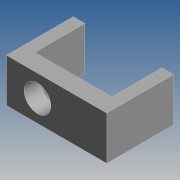
# Autodesk Inventor part: support_Servo
Saved by Autodesk Inventor 2017 (Build 210142000, 142)
## iProperties
Created: 2018-10-05
Part Number: support_Servo
Material: Générique
Document SubType Name: Modeling
Designer: Gilles Mottiez
Density: 1 g/cm^3
Appearance: Par défaut
Author: Gilles Mottiez
Autodesk Inventor part; units mm, degrees
ref_plane "YZ Plane" through (0, 0, 0) normal (1, 0, 0) x (0, 1, 0)
ref_plane "XZ Plane" through (0, 0, 0) normal (0, 1, 0) x (-1, 0, 0)
ref_plane "XY Plane" through (0, 0, 0) normal (0, 0, 1) x (1, 0, 0)
sketch "Sketch1" plane through (0, 0, 0) normal (0, 0, 1) x (1, 0, 0)
  line L0 (0, 0) -> (30, 0) construction
  line L1 (30, 0) -> (30, -20) construction
  line L2 (30, -20) -> (0, -20) construction
  line L3 (0, -20) -> (0, 0) construction
  line L4 (3.5, 0) -> (26.5, 0) construction
  line L5 (26.5, 0) -> (26.5, -15) construction
  line L6 (26.5, -15) -> (3.5, -15) construction
  line L7 (3.5, -15) -> (3.5, 0) construction
  line L8 (3.5, 0) -> (0, 0)
  line L9 (0, 0) -> (0, -20)
  line L10 (0, -20) -> (30, -20)
  line L11 (30, -20) -> (30, 0)
  line L12 (30, 0) -> (26.5, 0)
  line L13 (26.5, 0) -> (26.5, -15)
  line L14 (26.5, -15) -> (3.5, -15)
  line L15 (3.5, -15) -> (3.5, 0)
  point P0 (15, -15)
  point P1 (15, 0)
  dimension "d0" = 30
  dimension "d1" = 20
  dimension "d2" = 23
  dimension "d3" = 15
  constraints: 32 end point, 6 collinear, 4 parallel, 4 perpendicular, 2 horizontal, 2 midpoint, 1 point on line, 1 vertical alignment
  measures "d0" distance of L0.start L0.end
  measures "d1" distance of L2.end L0.start
  measures "d2" distance of L5.end L6.end
  measures "d3" distance of L4.end L5.end
extrude "Extrusion1" add sketch "Sketch1" along normal blind 13
sketch "Esquisse2" plane through (3.5, -15, 0) normal (0, 1, 0) x (1, 0, 0)
  line L0 (0, 0) -> (23, 0) construction
  line L1 (0, 0) -> (0, -13) construction
  line L2 (23, -13) -> (0, -13) construction
  line L3 (23, 0) -> (23, -13) construction
  circle A0 centre (5.8, -6.5) radius 4
  line L4 (0, 0) -> (0, -13) projected
  point P0 (-3.5, 0)
  point P1 (0, -6.5)
  dimension "d6" = 8
  dimension "d7" = 5.8
  constraints: 1 centre point, 1 horizontal alignment, 1 midpoint
  measures "d6" diameter of A0
  measures "d7" distance from line of L1 A0.centre
extrude "Extrusion2" cut sketch "Esquisse2" against normal through all
